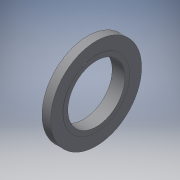
# Autodesk Inventor part: A1-19027-400-06 ALTERNATE TEST FLANGE
Saved by Autodesk Inventor 2017.3 (Build 213257000, 257)
## iProperties
Created: 2020-03-10
Part Number: A1-19027-400-06 ALTERNATE TEST FLANGE
Material: Generic
Document SubType Name: Modeling
Designer: BEM
Density: 1 g/cm^3
Appearance: Default
Author: BEM
Autodesk Inventor part; units mm, degrees
ref_plane "YZ Plane" through (0, 0, 0) normal (1, 0, 0) x (0, 1, 0)
ref_plane "XZ Plane" through (0, 0, 0) normal (0, 1, 0) x (-1, 0, 0)
ref_plane "XY Plane" through (0, 0, 0) normal (0, 0, 1) x (1, 0, 0)
sketch "Sketch1" plane through (0, 0, 0) normal (0, 0, 1) x (1, 0, 0)
  line L0 (0, 0) -> (0, 163.576)
  line L1 (0, 163.576) -> (-73.2155, 163.576)
  line L2 (-73.2155, 163.576) -> (-73.2155, 187.325)
  line L3 (-73.2155, 187.325) -> (-50.8635, 187.325)
  line L4 (-50.8635, 187.325) -> (-50.8635, 260.35)
  line L5 (0, 190.5) -> (0, 163.576)
  line L6 (-50.8635, 260.35) -> (-1.5875, 260.35)
  line L7 (-1.5875, 260.35) -> (-1.5875, 190.5)
  line L8 (-1.5875, 190.5) -> (0, 190.5)
  line L9 (-87.8586, 0) -> (14.6431, 0) projected
  dimension "d0" = 1.5875
  dimension "d2" = 49.276
  dimension "d3" = 260.35
  dimension "d4" = 190.5
  dimension "d5" = 163.576
  dimension "d6" = 187.325
  dimension "d7" = 71.628
  dimension "d8" = 90
  constraints: 18 end point, 4 perpendicular, 1 horizontal, 1 parallel, 1 point on line, 1 vertical
  measures "d0" distance between parallel lines of L7 L5
  measures "d2" distance between parallel lines of L7 L4
  measures "d3" distance from line of L0.start L6
  measures "d4" distance of L5.start L0.start
  measures "d5" distance from line of L0.start L1
  measures "d6" vertical distance of L0.start L3.end
  measures "d7" distance between parallel lines of L2 L7
  measures "d8" angle of L3 L4
revolve "Revolution1" add sketch "Sketch1" angle 360 about axis through (-10, 0, 0) along (1, 0, 0)
sketch "Sketch2" plane through (0, 0, 0) normal (0, 0, 1) x (1, 0, 0)
  line L0 (-73.2155, -187.325) -> (-73.2155, -163.576) projected
  line L1 (-73.2155, -163.576) -> (0, -163.576) projected
  line L2 (0, -163.576) -> (0, -190.5) projected
  line L3 (0, -190.5) -> (-1.5875, -190.5) projected
  line L4 (-1.5875, -190.5) -> (-1.5875, -260.35) projected
  line L5 (-1.5875, -260.35) -> (-50.8635, -260.35) projected
  line L6 (-50.8635, -260.35) -> (-50.8635, -187.325) projected
  line L7 (-50.8635, -187.325) -> (-73.2155, -187.325) projected
  line L8 (-73.2155, 163.576) -> (-73.2155, 187.325) projected
  line L9 (-73.2155, 187.325) -> (-50.8635, 187.325) projected
  line L10 (-50.8635, 187.325) -> (-50.8635, 260.35) projected
  line L11 (-50.8635, 260.35) -> (-1.5875, 260.35) projected
  line L12 (-1.5875, 260.35) -> (-1.5875, 190.5) projected
  line L13 (-1.5875, 190.5) -> (0, 190.5) projected
  line L14 (0, 190.5) -> (0, 163.576) projected
  line L15 (0, 163.576) -> (-73.2155, 163.576) projected
  line L16 (0, -190.5) -> (0, 190.5) projected
  line L17 (0, 165.1) -> (-25.4, 165.1)
  line L18 (-73.2155, 165.1) -> (-73.2155, 166.6875)
  line L19 (-73.2155, 166.6875) -> (-64.6886, 177.8)
  line L20 (-64.6886, 177.8) -> (-60.3885, 177.8)
  line L21 (-50.8635, 177.8) -> (-50.8635, 187.325) construction
  line L22 (0, 165.1) -> (-25.4, 165.1) construction
  line L23 (-25.4, 165.1) -> (-25.4, 160.3375)
  line L24 (-25.4, 160.3375) -> (0, 160.3375)
  line L25 (0, 160.3375) -> (0, 165.1)
  arc A0 (-60.3885, 177.8) -> (-50.8635, 187.325) centre (-60.3885, 187.325) ccw
  line L26 (-60.3885, 177.8) -> (-50.8635, 177.8) construction
  line L27 (-25.4, 165.1) -> (-73.2155, 165.1)
  line L28 (-50.8635, -260.35) -> (-50.8635, 260.35) projected
  line L29 (-50.8635, 187.325) -> (-50.8635, 260.35)
  line L30 (-50.8635, 260.35) -> (-1.5875, 260.35)
  line L31 (-1.5875, 190.5) -> (0, 190.5)
  line L32 (-87.8586, 0) -> (14.6431, 0) projected
  point P0 (0, 0)
  dimension "d10" = 1.5875
  dimension "d11" = 37.5
  dimension "d12" = 177.8
  dimension "d13" = 25.4
  dimension "d14" = 160.3375
  dimension "d15" = 165.1
  dimension "d16" = 22.225
  constraints: 28 end point, 7 parallel, 5 perpendicular, 3 horizontal, 3 tangent, 2 collinear, 2 point on circle, 2 point on line, 1 centre point
  measures "d10" distance of L18.start L18.end
  measures "d11" angle of L8 L19
  measures "d12" distance from line of point (0, 0) L20
  measures "d13" distance between parallel lines of L23 L16
  measures "d14" distance from line of point (0, 0) L24
  measures "d15" distance from line of point (0, 0) L17
  measures "d16" distance from line of L9.end L17
revolve "Revolution2" cut sketch "Sketch2" angle 360 about axis through (-10, 0, 0) along (1, 0, 0) contours A0 L20 L19 L8 L9
body "Solid1"
